Autodesk Fusion 360 part; units mm, degrees
(part 3 of 5)
sketch "midlayer" plane through (0, 0, 0) normal (0, 0, -1) x (1, 0, 0)
  line L0 (154.732, -58.8215) -> (154.732, -59.8219)
  line L1 (154.732, -59.8219) -> (140.732, -59.8219)
  line L2 (140.732, -59.8219) -> (140.732, -58.8215)
  line L3 (140.732, -58.8215) -> (139.931, -58.8215)
  line L4 (139.931, -58.8215) -> (139.931, -55.7223)
  line L5 (139.931, -55.7223) -> (140.732, -55.7223)
  line L6 (140.732, -55.7223) -> (140.732, -49.9223)
  line L7 (140.732, -49.9223) -> (139.931, -49.9223)
  line L8 (139.931, -49.9223) -> (139.931, -46.8217)
  line L9 (139.931, -46.8217) -> (140.732, -46.8217)
  line L10 (140.732, -46.8217) -> (140.732, -45.8227)
  line L11 (140.732, -45.8227) -> (154.732, -45.8227)
  line L12 (154.732, -45.8227) -> (154.732, -46.8217)
  line L13 (154.732, -46.8217) -> (155.531, -46.8217)
  line L14 (155.531, -46.8217) -> (155.531, -49.9223)
  line L15 (155.531, -49.9223) -> (154.732, -49.9223)
  line L16 (154.732, -49.9223) -> (154.732, -55.7223)
  line L17 (154.732, -55.7223) -> (155.531, -55.7223)
  line L18 (155.531, -55.7223) -> (155.531, -58.8215)
  line L19 (155.531, -58.8215) -> (154.732, -58.8215)
  line L20 (116.632, -46.8217) -> (117.431, -46.8217)
  line L21 (117.431, -46.8217) -> (117.431, -49.9223)
  line L22 (117.431, -49.9223) -> (116.632, -49.9223)
  line L23 (116.632, -49.9223) -> (116.632, -55.7223)
  line L24 (116.632, -55.7223) -> (117.431, -55.7223)
  line L25 (117.431, -55.7223) -> (117.431, -58.8215)
  line L26 (117.431, -58.8215) -> (116.632, -58.8215)
  line L27 (116.632, -58.8215) -> (116.632, -59.8219)
  line L28 (116.632, -59.8219) -> (102.632, -59.8219)
  line L29 (102.632, -59.8219) -> (102.632, -58.8215)
  line L30 (102.632, -58.8215) -> (101.831, -58.8215)
  line L31 (101.831, -58.8215) -> (101.831, -55.7223)
  line L32 (101.831, -55.7223) -> (102.632, -55.7223)
  line L33 (102.632, -55.7223) -> (102.632, -49.9223)
  line L34 (102.632, -49.9223) -> (101.831, -49.9223)
  line L35 (101.831, -49.9223) -> (101.831, -46.8217)
  line L36 (101.831, -46.8217) -> (102.632, -46.8217)
  line L37 (102.632, -46.8217) -> (102.632, -45.8227)
  line L38 (102.632, -45.8227) -> (116.632, -45.8227)
  line L39 (116.632, -45.8227) -> (116.632, -46.8217)
  line L40 (192.832, -59.8219) -> (178.832, -59.8219)
  line L41 (178.832, -59.8219) -> (178.832, -58.8215)
  line L42 (178.832, -58.8215) -> (178.031, -58.8215)
  line L43 (178.031, -58.8215) -> (178.031, -55.7223)
  line L44 (178.031, -55.7223) -> (178.832, -55.7223)
  line L45 (178.832, -55.7223) -> (178.832, -49.9223)
  line L46 (178.832, -49.9223) -> (178.031, -49.9223)
  line L47 (178.031, -49.9223) -> (178.031, -46.8217)
  line L48 (178.031, -46.8217) -> (178.832, -46.8217)
  line L49 (178.832, -46.8217) -> (178.832, -45.8227)
  line L50 (178.832, -45.8227) -> (192.832, -45.8227)
  line L51 (192.832, -45.8227) -> (192.832, -46.8217)
  line L52 (192.832, -46.8217) -> (193.631, -46.8217)
  line L53 (193.631, -46.8217) -> (193.631, -49.9223)
  line L54 (193.631, -49.9223) -> (192.832, -49.9223)
  line L55 (192.832, -49.9223) -> (192.832, -55.7223)
  line L56 (192.832, -55.7223) -> (193.631, -55.7223)
  line L57 (193.631, -55.7223) -> (193.631, -58.8215)
  line L58 (193.631, -58.8215) -> (192.832, -58.8215)
  line L59 (192.832, -58.8215) -> (192.832, -59.8219)
  line L60 (76.1503, -36.6737) -> (76.9511, -36.6737)
  line L61 (76.9511, -36.6737) -> (76.9511, -39.7715)
  line L62 (76.9511, -39.7715) -> (76.1503, -39.7715)
  line L63 (76.1503, -39.7715) -> (76.1503, -40.7719)
  line L64 (76.1503, -40.7719) -> (62.151, -40.7719)
  line L65 (62.151, -40.7719) -> (62.151, -39.7715)
  line L66 (62.151, -39.7715) -> (61.3502, -39.7715)
  line L67 (61.3502, -39.7715) -> (61.3502, -36.6737)
  line L68 (61.3502, -36.6737) -> (62.151, -36.6737)
  line L69 (62.151, -36.6737) -> (62.151, -30.8722)
  line L70 (62.151, -30.8722) -> (61.3502, -30.8722)
  line L71 (61.3502, -30.8722) -> (61.3502, -27.7716)
  line L72 (61.3502, -27.7716) -> (62.151, -27.7716)
  line L73 (62.151, -27.7716) -> (62.151, -26.7725)
  line L74 (62.151, -26.7725) -> (76.1503, -26.7725)
  line L75 (76.1503, -26.7725) -> (76.1503, -27.7716)
  line L76 (76.1503, -27.7716) -> (76.9511, -27.7716)
  line L77 (76.9511, -27.7716) -> (76.9511, -30.8722)
  line L78 (76.9511, -30.8722) -> (76.1503, -30.8722)
  line L79 (76.1503, -30.8722) -> (76.1503, -36.6737)
  line L80 (130.919, -64.8727) -> (130.919, -65.8717)
  line L81 (130.919, -65.8717) -> (131.72, -65.8717)
  line L82 (131.72, -65.8717) -> (131.72, -68.9723)
  line L83 (131.72, -68.9723) -> (130.919, -68.9723)
  line L84 (130.919, -68.9723) -> (130.919, -74.7723)
  line L85 (130.919, -74.7723) -> (131.72, -74.7723)
  line L86 (131.72, -74.7723) -> (131.72, -77.8715)
  line L87 (131.72, -77.8715) -> (130.919, -77.8715)
  line L88 (130.919, -77.8715) -> (130.919, -78.8719)
  line L89 (130.919, -78.8719) -> (116.92, -78.8719)
  line L90 (116.92, -78.8719) -> (116.92, -77.8715)
  line L91 (116.92, -77.8715) -> (116.119, -77.8715)
  line L92 (116.119, -77.8715) -> (116.119, -74.7723)
  line L93 (116.119, -74.7723) -> (116.92, -74.7723)
  line L94 (116.92, -74.7723) -> (116.92, -68.9723)
  line L95 (116.92, -68.9723) -> (116.119, -68.9723)
  line L96 (116.119, -68.9723) -> (116.119, -65.8717)
  line L97 (116.119, -65.8717) -> (116.92, -65.8717)
  line L98 (116.92, -65.8717) -> (116.92, -64.8727)
  line L99 (116.92, -64.8727) -> (130.919, -64.8727)
  line L100 (169.019, -68.9723) -> (169.019, -74.7723)
  line L101 (169.019, -74.7723) -> (169.82, -74.7723)
  line L102 (169.82, -74.7723) -> (169.82, -77.8715)
  line L103 (169.82, -77.8715) -> (169.019, -77.8715)
  line L104 (169.019, -77.8715) -> (169.019, -78.8719)
  line L105 (169.019, -78.8719) -> (155.02, -78.8719)
  line L106 (155.02, -78.8719) -> (155.02, -77.8715)
  line L107 (155.02, -77.8715) -> (154.219, -77.8715)
  line L108 (154.219, -77.8715) -> (154.219, -74.7723)
  line L109 (154.219, -74.7723) -> (155.02, -74.7723)
  line L110 (155.02, -74.7723) -> (155.02, -68.9723)
  line L111 (155.02, -68.9723) -> (154.219, -68.9723)
  line L112 (154.219, -68.9723) -> (154.219, -65.8717)
  line L113 (154.219, -65.8717) -> (155.02, -65.8717)
  line L114 (155.02, -65.8717) -> (155.02, -64.8727)
  line L115 (155.02, -64.8727) -> (169.019, -64.8727)
  line L116 (169.019, -64.8727) -> (169.019, -65.8717)
  line L117 (169.019, -65.8717) -> (169.82, -65.8717)
  line L118 (169.82, -65.8717) -> (169.82, -68.9723)
  line L119 (169.82, -68.9723) -> (169.019, -68.9723)
  arc A0 (54.0504, -25.8024) -> (53.0504, -26.8024) centre (54.0504, -26.8024) ccw
  line L120 (54.0504, -25.8024) -> (59.6225, -25.8024)
  arc A1 (60.6225, -26.8024) -> (59.6225, -25.8024) centre (59.6225, -26.8024) ccw
  line L121 (60.6225, -26.8024) -> (60.6225, -38.3016)
  arc A2 (59.6225, -39.3016) -> (60.6225, -38.3016) centre (59.6225, -38.3016) ccw
  line L122 (59.6225, -39.3016) -> (54.0504, -39.3016)
  arc A3 (53.0504, -38.3016) -> (54.0504, -39.3016) centre (54.0504, -38.3016) ccw
  line L123 (53.0504, -38.3016) -> (53.0504, -26.8024)
  line L124 (219.025, -17.6237) -> (219.826, -17.6237)
  line L125 (219.826, -17.6237) -> (219.826, -20.7216)
  line L126 (219.826, -20.7216) -> (219.025, -20.7216)
  line L127 (219.025, -20.7216) -> (219.025, -21.722)
  line L128 (219.025, -21.722) -> (205.026, -21.722)
  line L129 (205.026, -21.722) -> (205.026, -20.7216)
  line L130 (205.026, -20.7216) -> (204.225, -20.7216)
  line L131 (204.225, -20.7216) -> (204.225, -17.6237)
  line L132 (204.225, -17.6237) -> (205.026, -17.6237)
  line L133 (205.026, -17.6237) -> (205.026, -11.8222)
  line L134 (205.026, -11.8222) -> (204.225, -11.8222)
  line L135 (204.225, -11.8222) -> (204.225, -8.7216)
  line L136 (204.225, -8.7216) -> (205.026, -8.7216)
  line L137 (205.026, -8.7216) -> (205.026, -7.7225)
  line L138 (205.026, -7.7225) -> (219.025, -7.7225)
  line L139 (219.025, -7.7225) -> (219.025, -8.7216)
  line L140 (219.025, -8.7216) -> (219.826, -8.7216)
  line L141 (219.826, -8.7216) -> (219.826, -11.8222)
  line L142 (219.826, -11.8222) -> (219.025, -11.8222)
  line L143 (219.025, -11.8222) -> (219.025, -17.6237)
  line L144 (150.77, -65.8717) -> (150.77, -68.9723)
  line L145 (150.77, -68.9723) -> (149.969, -68.9723)
  line L146 (149.969, -68.9723) -> (149.969, -74.7723)
  line L147 (149.969, -74.7723) -> (150.77, -74.7723)
  line L148 (150.77, -74.7723) -> (150.77, -77.8715)
  line L149 (150.77, -77.8715) -> (149.969, -77.8715)
  line L150 (149.969, -77.8715) -> (149.969, -78.8719)
  line L151 (149.969, -78.8719) -> (135.97, -78.8719)
  line L152 (135.97, -78.8719) -> (135.97, -77.8715)
  line L153 (135.97, -77.8715) -> (135.169, -77.8715)
  line L154 (135.169, -77.8715) -> (135.169, -74.7723)
  line L155 (135.169, -74.7723) -> (135.97, -74.7723)
  line L156 (135.97, -74.7723) -> (135.97, -68.9723)
  line L157 (135.97, -68.9723) -> (135.169, -68.9723)
  line L158 (135.169, -68.9723) -> (135.169, -65.8717)
  line L159 (135.169, -65.8717) -> (135.97, -65.8717)
  line L160 (135.97, -65.8717) -> (135.97, -64.8727)
  line L161 (135.97, -64.8727) -> (149.969, -64.8727)
  line L162 (149.969, -64.8727) -> (149.969, -65.8717)
  line L163 (149.969, -65.8717) -> (150.77, -65.8717)
  line L164 (119.725, -19.2517) -> (119.725, -7.7524)
  arc A4 (120.725, -6.7524) -> (119.725, -7.7524) centre (120.725, -7.7524) ccw
  line L165 (120.725, -6.7524) -> (131.063, -6.7524)
  arc A5 (132.063, -7.7524) -> (131.063, -6.7524) centre (131.063, -7.7524) ccw
  line L166 (132.063, -7.7524) -> (132.063, -19.2517)
  arc A6 (131.063, -20.2517) -> (132.063, -19.2517) centre (131.063, -19.2517) ccw
  line L167 (131.063, -20.2517) -> (120.725, -20.2517)
  arc A7 (119.725, -19.2517) -> (120.725, -20.2517) centre (120.725, -19.2517) ccw
  line L168 (307.132, -36.6723) -> (307.931, -36.6723)
  line L169 (307.931, -36.6723) -> (307.931, -39.7715)
  line L170 (307.931, -39.7715) -> (307.132, -39.7715)
  line L171 (307.132, -39.7715) -> (307.132, -40.7719)
  line L172 (307.132, -40.7719) -> (293.132, -40.7719)
  line L173 (293.132, -40.7719) -> (293.132, -39.7715)
  line L174 (293.132, -39.7715) -> (292.331, -39.7715)
  line L175 (292.331, -39.7715) -> (292.331, -36.6723)
  line L176 (292.331, -36.6723) -> (293.132, -36.6723)
  line L177 (293.132, -36.6723) -> (293.132, -30.8722)
  line L178 (293.132, -30.8722) -> (292.331, -30.8722)
  line L179 (292.331, -30.8722) -> (292.331, -27.7716)
  line L180 (292.331, -27.7716) -> (293.132, -27.7716)
  line L181 (293.132, -27.7716) -> (293.132, -26.7725)
  line L182 (293.132, -26.7725) -> (307.132, -26.7725)
  line L183 (307.132, -26.7725) -> (307.132, -27.7716)
  line L184 (307.132, -27.7716) -> (307.931, -27.7716)
  line L185 (307.931, -27.7716) -> (307.931, -30.8722)
  line L186 (307.931, -30.8722) -> (307.132, -30.8722)
  line L187 (307.132, -30.8722) -> (307.132, -36.6723)
  line L188 (185.688, -17.6237) -> (186.487, -17.6237)
  line L189 (186.487, -17.6237) -> (186.487, -20.7216)
  line L190 (186.487, -20.7216) -> (185.688, -20.7216)
  line L191 (185.688, -20.7216) -> (185.688, -21.722)
  line L192 (185.688, -21.722) -> (166.926, -21.722)
  line L193 (166.926, -21.722) -> (166.926, -20.7216)
  line L194 (166.926, -20.7216) -> (166.125, -20.7216)
  line L195 (166.125, -20.7216) -> (166.125, -17.6237)
  line L196 (166.125, -17.6237) -> (166.926, -17.6237)
  line L197 (166.926, -17.6237) -> (166.926, -11.8222)
  line L198 (166.926, -11.8222) -> (166.125, -11.8222)
  line L199 (166.125, -11.8222) -> (166.125, -8.7216)
  line L200 (166.125, -8.7216) -> (166.926, -8.7216)
  line L201 (166.926, -8.7216) -> (166.926, -7.7225)
  line L202 (166.926, -7.7225) -> (185.688, -7.7225)
  line L203 (185.688, -7.7225) -> (185.688, -8.7216)
  line L204 (185.688, -8.7216) -> (186.487, -8.7216)
  line L205 (186.487, -8.7216) -> (186.487, -11.8222)
  line L206 (186.487, -11.8222) -> (185.688, -11.8222)
  line L207 (185.688, -11.8222) -> (185.688, -17.6237)
  line L208 (147.588, -17.6237) -> (148.387, -17.6237)
  line L209 (148.387, -17.6237) -> (148.387, -20.7216)
  line L210 (148.387, -20.7216) -> (147.588, -20.7216)
  line L211 (147.588, -20.7216) -> (147.588, -21.722)
  line L212 (147.588, -21.722) -> (133.587, -21.722)
  line L213 (133.587, -21.722) -> (133.587, -20.7216)
  line L214 (133.587, -20.7216) -> (132.788, -20.7216)
  line L215 (132.788, -20.7216) -> (132.788, -17.6237)
  line L216 (132.788, -17.6237) -> (133.587, -17.6237)
  line L217 (133.587, -17.6237) -> (133.587, -11.8222)
  line L218 (133.587, -11.8222) -> (132.788, -11.8222)
  line L219 (132.788, -11.8222) -> (132.788, -8.7216)
  line L220 (132.788, -8.7216) -> (133.587, -8.7216)
  line L221 (133.587, -8.7216) -> (133.587, -7.7225)
  line L222 (133.587, -7.7225) -> (147.588, -7.7225)
  line L223 (147.588, -7.7225) -> (147.588, -8.7216)
  line L224 (147.588, -8.7216) -> (148.387, -8.7216)
  line L225 (148.387, -8.7216) -> (148.387, -11.8222)
  line L226 (148.387, -11.8222) -> (147.588, -11.8222)
  line L227 (147.588, -11.8222) -> (147.588, -17.6237)
  arc A8 (84.2847, -39.3016) -> (85.2847, -38.3016) centre (84.2847, -38.3016) ccw
  line L228 (84.2847, -39.3016) -> (78.676, -39.3016)
  arc A9 (77.676, -38.3016) -> (78.676, -39.3016) centre (78.676, -38.3016) ccw
  line L229 (77.676, -38.3016) -> (77.676, -26.8024)
  arc A10 (78.676, -25.8024) -> (77.676, -26.8024) centre (78.676, -26.8024) ccw
  line L230 (78.676, -25.8024) -> (84.2847, -25.8024)
  arc A11 (85.2847, -26.8024) -> (84.2847, -25.8024) centre (84.2847, -26.8024) ccw
  line L231 (85.2847, -26.8024) -> (85.2847, -38.3016)
  line L232 (97.8697, -65.8717) -> (97.8697, -64.8727)
  line L233 (97.8697, -64.8727) -> (111.869, -64.8727)
  line L234 (111.869, -64.8727) -> (111.869, -65.8717)
  line L235 (111.869, -65.8717) -> (112.67, -65.8717)
  line L236 (112.67, -65.8717) -> (112.67, -68.9723)
  line L237 (112.67, -68.9723) -> (111.869, -68.9723)
  line L238 (111.869, -68.9723) -> (111.869, -74.7723)
  line L239 (111.869, -74.7723) -> (112.67, -74.7723)
  line L240 (112.67, -74.7723) -> (112.67, -77.8715)
  line L241 (112.67, -77.8715) -> (111.869, -77.8715)
  line L242 (111.869, -77.8715) -> (111.869, -78.8719)
  line L243 (111.869, -78.8719) -> (97.8697, -78.8719)
  line L244 (97.8697, -78.8719) -> (97.8697, -77.8715)
  line L245 (97.8697, -77.8715) -> (97.0689, -77.8715)
  line L246 (97.0689, -77.8715) -> (97.0689, -74.7723)
  line L247 (97.0689, -74.7723) -> (97.8697, -74.7723)
  line L248 (97.8697, -74.7723) -> (97.8697, -68.9723)
  line L249 (97.8697, -68.9723) -> (97.0689, -68.9723)
  line L250 (97.0689, -68.9723) -> (97.0689, -65.8717)
  line L251 (97.0689, -65.8717) -> (97.8697, -65.8717)
  line L252 (212.17, -77.8715) -> (211.369, -77.8715)
  line L253 (211.369, -77.8715) -> (211.369, -74.7723)
  line L254 (211.369, -74.7723) -> (212.17, -74.7723)
  line L255 (212.17, -74.7723) -> (212.17, -68.9723)
  line L256 (212.17, -68.9723) -> (211.369, -68.9723)
  line L257 (211.369, -68.9723) -> (211.369, -65.8717)
  line L258 (211.369, -65.8717) -> (212.17, -65.8717)
  line L259 (212.17, -65.8717) -> (212.17, -64.8727)
  line L260 (212.17, -64.8727) -> (226.169, -64.8727)
  line L261 (226.169, -64.8727) -> (226.169, -65.8717)
  line L262 (226.169, -65.8717) -> (226.97, -65.8717)
  line L263 (226.97, -65.8717) -> (226.97, -68.9723)
  line L264 (226.97, -68.9723) -> (226.169, -68.9723)
  line L265 (226.169, -68.9723) -> (226.169, -74.7723)
  line L266 (226.169, -74.7723) -> (226.97, -74.7723)
  line L267 (226.97, -74.7723) -> (226.97, -77.8715)
  line L268 (226.97, -77.8715) -> (226.169, -77.8715)
  line L269 (226.169, -77.8715) -> (226.169, -78.8719)
  line L270 (226.169, -78.8719) -> (212.17, -78.8719)
  line L271 (212.17, -78.8719) -> (212.17, -77.8715)
  arc A12 (154.863, -20.2517) -> (155.863, -19.2517) centre (154.863, -19.2517) ccw
  line L272 (154.863, -20.2517) -> (150.112, -20.2517)
  arc A13 (149.112, -19.2517) -> (150.112, -20.2517) centre (150.112, -19.2517) ccw
  line L273 (149.112, -19.2517) -> (149.112, -7.7524)
  arc A14 (150.112, -6.7524) -> (149.112, -7.7524) centre (150.112, -7.7524) ccw
  line L274 (150.112, -6.7524) -> (154.863, -6.7524)
  arc A15 (155.863, -7.7524) -> (154.863, -6.7524) centre (154.863, -7.7524) ccw
  line L275 (155.863, -7.7524) -> (155.863, -19.2517)
  arc A16 (220.551, -19.2517) -> (221.551, -20.2517) centre (221.551, -19.2517) ccw
  line L276 (220.551, -19.2517) -> (220.551, -7.7524)
  arc A17 (221.551, -6.7524) -> (220.551, -7.7524) centre (221.551, -7.7524) ccw
  line L277 (221.551, -6.7524) -> (227.126, -6.7524)
  arc A18 (228.126, -7.7524) -> (227.126, -6.7524) centre (227.126, -7.7524) ccw
  line L278 (228.126, -7.7524) -> (228.126, -19.2517)
  arc A19 (227.126, -20.2517) -> (228.126, -19.2517) centre (227.126, -19.2517) ccw
  line L279 (227.126, -20.2517) -> (221.551, -20.2517)
  line L280 (284.032, -38.3016) -> (284.032, -26.8024)
  arc A20 (285.032, -25.8024) -> (284.032, -26.8024) centre (285.032, -26.8024) ccw
  line L281 (285.032, -25.8024) -> (290.607, -25.8024)
  arc A21 (291.607, -26.8024) -> (290.607, -25.8024) centre (290.607, -26.8024) ccw
  line L282 (291.607, -26.8024) -> (291.607, -38.3016)
  arc A22 (290.607, -39.3016) -> (291.607, -38.3016) centre (290.607, -38.3016) ccw
  line L283 (290.607, -39.3016) -> (285.032, -39.3016)
  arc A23 (284.032, -38.3016) -> (285.032, -39.3016) centre (285.032, -38.3016) ccw
  arc A24 (309.657, -25.8024) -> (308.657, -26.8024) centre (309.657, -26.8024) ccw
  line L284 (309.657, -25.8024) -> (315.248, -25.8024)
  arc A25 (316.248, -26.8024) -> (315.248, -25.8024) centre (315.248, -26.8024) ccw
  line L285 (316.248, -26.8024) -> (316.248, -38.3016)
  arc A26 (315.248, -39.3016) -> (316.248, -38.3016) centre (315.248, -38.3016) ccw
  line L286 (315.248, -39.3016) -> (309.657, -39.3016)
  arc A27 (308.657, -38.3016) -> (309.657, -39.3016) centre (309.657, -38.3016) ccw
  line L287 (308.657, -38.3016) -> (308.657, -26.8024)
  line L288 (319.038, -55.7223) -> (319.837, -55.7223)
  line L289 (319.837, -55.7223) -> (319.837, -58.8215)
  line L290 (319.837, -58.8215) -> (319.038, -58.8215)
  line L291 (319.038, -58.8215) -> (319.038, -59.8219)
  line L292 (319.038, -59.8219) -> (305.037, -59.8219)
  line L293 (305.037, -59.8219) -> (305.037, -58.8215)
  line L294 (305.037, -58.8215) -> (304.238, -58.8215)
  line L295 (304.238, -58.8215) -> (304.238, -55.7223)
  line L296 (304.238, -55.7223) -> (305.037, -55.7223)
  line L297 (305.037, -55.7223) -> (305.037, -49.9223)
  line L298 (305.037, -49.9223) -> (304.238, -49.9223)
  line L299 (304.238, -49.9223) -> (304.238, -46.8217)
  line L300 (304.238, -46.8217) -> (305.037, -46.8217)
  line L301 (305.037, -46.8217) -> (305.037, -45.8227)
  line L302 (305.037, -45.8227) -> (319.038, -45.8227)
  line L303 (319.038, -45.8227) -> (319.038, -46.8217)
  line L304 (319.038, -46.8217) -> (319.837, -46.8217)
  line L305 (319.837, -46.8217) -> (319.837, -49.9223)
  line L306 (319.837, -49.9223) -> (319.038, -49.9223)
  line L307 (319.038, -49.9223) -> (319.038, -55.7223)
  line L308 (303.513, -45.8525) -> (303.513, -57.3516)
  arc A28 (302.513, -58.3516) -> (303.513, -57.3516) centre (302.513, -57.3516) ccw
  line L309 (302.513, -58.3516) -> (296.938, -58.3516)
  arc A29 (295.938, -57.3516) -> (296.938, -58.3516) centre (296.938, -57.3516) ccw
  line L310 (295.938, -57.3516) -> (295.938, -45.8525)
  arc A30 (296.938, -44.8525) -> (295.938, -45.8525) centre (296.938, -45.8525) ccw
  line L311 (296.938, -44.8525) -> (302.513, -44.8525)
  arc A31 (303.513, -45.8525) -> (302.513, -44.8525) centre (302.513, -45.8525) ccw
  arc A32 (327.137, -58.3516) -> (328.137, -57.3516) centre (327.137, -57.3516) ccw
  line L312 (327.137, -58.3516) -> (321.562, -58.3516)
  arc A33 (320.562, -57.3516) -> (321.562, -58.3516) centre (321.562, -57.3516) ccw
  line L313 (320.562, -57.3516) -> (320.562, -45.8525)
  arc A34 (321.562, -44.8525) -> (320.562, -45.8525) centre (321.562, -45.8525) ccw
  line L314 (321.562, -44.8525) -> (327.137, -44.8525)
  arc A35 (328.137, -45.8525) -> (327.137, -44.8525) centre (327.137, -45.8525) ccw
  line L315 (328.137, -45.8525) -> (328.137, -57.3516)
  circle A36 centre (-4.6103, -105.1519) radius 1.55
  circle A37 centre (-4.6103, 4.27) radius 1.55
  circle A38 centre (371.512, -105.1519) radius 1.55
  circle A39 centre (371.512, 4.27) radius 1.55
  line L316 (174.07, -78.8719) -> (174.07, -77.8715)
  line L317 (174.07, -77.8715) -> (173.269, -77.8715)
  line L318 (173.269, -77.8715) -> (173.269, -74.7723)
  line L319 (173.269, -74.7723) -> (174.07, -74.7723)
  line L320 (174.07, -74.7723) -> (174.07, -68.9723)
  line L321 (174.07, -68.9723) -> (173.269, -68.9723)
  line L322 (173.269, -68.9723) -> (173.269, -65.8717)
  line L323 (173.269, -65.8717) -> (174.07, -65.8717)
  line L324 (174.07, -65.8717) -> (174.07, -64.8727)
  line L325 (174.07, -64.8727) -> (188.069, -64.8727)
  line L326 (188.069, -64.8727) -> (188.069, -65.8717)
  line L327 (188.069, -65.8717) -> (188.87, -65.8717)
  line L328 (188.87, -65.8717) -> (188.87, -68.9723)
  line L329 (188.87, -68.9723) -> (188.069, -68.9723)
  line L330 (188.069, -68.9723) -> (188.069, -74.7723)
  line L331 (188.069, -74.7723) -> (188.87, -74.7723)
  line L332 (188.87, -74.7723) -> (188.87, -77.8715)
  line L333 (188.87, -77.8715) -> (188.069, -77.8715)
  line L334 (188.069, -77.8715) -> (188.069, -78.8719)
  line L335 (188.069, -78.8719) -> (174.07, -78.8719)
  line L336 (207.119, -64.8727) -> (207.119, -65.8717)
  line L337 (207.119, -65.8717) -> (207.92, -65.8717)
  line L338 (207.92, -65.8717) -> (207.92, -68.9723)
  line L339 (207.92, -68.9723) -> (207.119, -68.9723)
  line L340 (207.119, -68.9723) -> (207.119, -74.7723)
  line L341 (207.119, -74.7723) -> (207.92, -74.7723)
  line L342 (207.92, -74.7723) -> (207.92, -77.8715)
  line L343 (207.92, -77.8715) -> (207.119, -77.8715)
  line L344 (207.119, -77.8715) -> (207.119, -78.8719)
  line L345 (207.119, -78.8719) -> (193.12, -78.8719)
  line L346 (193.12, -78.8719) -> (193.12, -77.8715)
  line L347 (193.12, -77.8715) -> (192.319, -77.8715)
  line L348 (192.319, -77.8715) -> (192.319, -74.7723)
  line L349 (192.319, -74.7723) -> (193.12, -74.7723)
  line L350 (193.12, -74.7723) -> (193.12, -68.9723)
  line L351 (193.12, -68.9723) -> (192.319, -68.9723)
  line L352 (192.319, -68.9723) -> (192.319, -65.8717)
  line L353 (192.319, -65.8717) -> (193.12, -65.8717)
  line L354 (193.12, -65.8717) -> (193.12, -64.8727)
  line L355 (193.12, -64.8727) -> (207.119, -64.8727)
  line L356 (182.794, -93.8223) -> (183.595, -93.8223)
  line L357 (183.595, -93.8223) -> (183.595, -88.0223)
  line L358 (183.595, -88.0223) -> (182.794, -88.0223)
  line L359 (182.794, -88.0223) -> (182.794, -84.9217)
  line L360 (182.794, -84.9217) -> (183.595, -84.9217)
  line L361 (183.595, -84.9217) -> (183.595, -83.9227)
  line L362 (183.595, -83.9227) -> (197.594, -83.9227)
  line L363 (197.594, -83.9227) -> (197.594, -84.9217)
  line L364 (197.594, -84.9217) -> (198.395, -84.9217)
  line L365 (198.395, -84.9217) -> (198.395, -88.0223)
  line L366 (198.395, -88.0223) -> (197.594, -88.0223)
  line L367 (197.594, -88.0223) -> (197.594, -93.8223)
  line L368 (197.594, -93.8223) -> (198.395, -93.8223)
  line L369 (198.395, -93.8223) -> (198.395, -96.9215)
  line L370 (198.395, -96.9215) -> (197.594, -96.9215)
  line L371 (197.594, -96.9215) -> (197.594, -97.9219)
  line L372 (197.594, -97.9219) -> (183.595, -97.9219)
  line L373 (183.595, -97.9219) -> (183.595, -96.9215)
  line L374 (183.595, -96.9215) -> (182.794, -96.9215)
  line L375 (182.794, -96.9215) -> (182.794, -93.8223)
  line L376 (201.844, -96.9215) -> (201.844, -93.8223)
  line L377 (201.844, -93.8223) -> (202.645, -93.8223)
  line L378 (202.645, -93.8223) -> (202.645, -88.0223)
  line L379 (202.645, -88.0223) -> (201.844, -88.0223)
  line L380 (201.844, -88.0223) -> (201.844, -84.9217)
  line L381 (201.844, -84.9217) -> (202.645, -84.9217)
  line L382 (202.645, -84.9217) -> (202.645, -83.9227)
  line L383 (202.645, -83.9227) -> (216.644, -83.9227)
  line L384 (216.644, -83.9227) -> (216.644, -84.9217)
  line L385 (216.644, -84.9217) -> (217.445, -84.9217)
  line L386 (217.445, -84.9217) -> (217.445, -88.0223)
  line L387 (217.445, -88.0223) -> (216.644, -88.0223)
  line L388 (216.644, -88.0223) -> (216.644, -93.8223)
  line L389 (216.644, -93.8223) -> (217.445, -93.8223)
  line L390 (217.445, -93.8223) -> (217.445, -96.9215)
  line L391 (217.445, -96.9215) -> (216.644, -96.9215)
  line L392 (216.644, -96.9215) -> (216.644, -97.9219)
  line L393 (216.644, -97.9219) -> (202.645, -97.9219)
  line L394 (202.645, -97.9219) -> (202.645, -96.9215)
  line L395 (202.645, -96.9215) -> (201.844, -96.9215)
  line L396 (220.894, -84.9217) -> (221.695, -84.9217)
  line L397 (221.695, -84.9217) -> (221.695, -83.9227)
  line L398 (221.695, -83.9227) -> (235.694, -83.9227)
  line L399 (235.694, -83.9227) -> (235.694, -84.9217)
  line L400 (235.694, -84.9217) -> (236.495, -84.9217)
  line L401 (236.495, -84.9217) -> (236.495, -88.0223)
  line L402 (236.495, -88.0223) -> (235.694, -88.0223)
  line L403 (235.694, -88.0223) -> (235.694, -93.8223)
  line L404 (235.694, -93.8223) -> (236.495, -93.8223)
  line L405 (236.495, -93.8223) -> (236.495, -96.9215)
  line L406 (236.495, -96.9215) -> (235.694, -96.9215)
  line L407 (235.694, -96.9215) -> (235.694, -97.9219)
  line L408 (235.694, -97.9219) -> (221.695, -97.9219)
  line L409 (221.695, -97.9219) -> (221.695, -96.9215)
  line L410 (221.695, -96.9215) -> (220.894, -96.9215)
  line L411 (220.894, -96.9215) -> (220.894, -93.8223)
  line L412 (220.894, -93.8223) -> (221.695, -93.8223)
  line L413 (221.695, -93.8223) -> (221.695, -88.0223)
  line L414 (221.695, -88.0223) -> (220.894, -88.0223)
  line L415 (220.894, -88.0223) -> (220.894, -84.9217)
  line L416 (254.744, -97.9219) -> (240.745, -97.9219)
  line L417 (240.745, -97.9219) -> (240.745, -96.9215)
  line L418 (240.745, -96.9215) -> (239.944, -96.9215)
  line L419 (239.944, -96.9215) -> (239.944, -93.8223)
  line L420 (239.944, -93.8223) -> (240.745, -93.8223)
  line L421 (240.745, -93.8223) -> (240.745, -88.0223)
  line L422 (240.745, -88.0223) -> (239.944, -88.0223)
  line L423 (239.944, -88.0223) -> (239.944, -84.9217)
  line L424 (239.944, -84.9217) -> (240.745, -84.9217)
  line L425 (240.745, -84.9217) -> (240.745, -83.9227)
  line L426 (240.745, -83.9227) -> (254.744, -83.9227)
  line L427 (254.744, -83.9227) -> (254.744, -84.9217)
  line L428 (254.744, -84.9217) -> (255.545, -84.9217)
  line L429 (255.545, -84.9217) -> (255.545, -88.0223)
  line L430 (255.545, -88.0223) -> (254.744, -88.0223)
  line L431 (254.744, -88.0223) -> (254.744, -93.8223)
  line L432 (254.744, -93.8223) -> (255.545, -93.8223)
  line L433 (255.545, -93.8223) -> (255.545, -96.9215)
  line L434 (255.545, -96.9215) -> (254.744, -96.9215)
  line L435 (254.744, -96.9215) -> (254.744, -97.9219)
  line L436 (144.694, -88.0223) -> (144.694, -84.9217)
  line L437 (144.694, -84.9217) -> (145.495, -84.9217)
  line L438 (145.495, -84.9217) -> (145.495, -83.9227)
  line L439 (145.495, -83.9227) -> (159.494, -83.9227)
  line L440 (159.494, -83.9227) -> (159.494, -84.9217)
  line L441 (159.494, -84.9217) -> (160.295, -84.9217)
  line L442 (160.295, -84.9217) -> (160.295, -88.0223)
  line L443 (160.295, -88.0223) -> (159.494, -88.0223)
  line L444 (159.494, -88.0223) -> (159.494, -93.8223)
  line L445 (159.494, -93.8223) -> (160.295, -93.8223)
  line L446 (160.295, -93.8223) -> (160.295, -96.9215)
  line L447 (160.295, -96.9215) -> (159.494, -96.9215)
  line L448 (159.494, -96.9215) -> (159.494, -97.9219)
  line L449 (159.494, -97.9219) -> (145.495, -97.9219)
  line L450 (145.495, -97.9219) -> (145.495, -96.9215)
  line L451 (145.495, -96.9215) -> (144.694, -96.9215)
  line L452 (144.694, -96.9215) -> (144.694, -93.8223)
  line L453 (144.694, -93.8223) -> (145.495, -93.8223)
  line L454 (145.495, -93.8223) -> (145.495, -88.0223)
  line L455 (145.495, -88.0223) -> (144.694, -88.0223)
  line L456 (164.545, -93.8223) -> (164.545, -88.0223)
  line L457 (164.545, -88.0223) -> (163.744, -88.0223)
  line L458 (163.744, -88.0223) -> (163.744, -84.9217)
  line L459 (163.744, -84.9217) -> (164.545, -84.9217)
  line L460 (164.545, -84.9217) -> (164.545, -83.9227)
  line L461 (164.545, -83.9227) -> (178.544, -83.9227)
  line L462 (178.544, -83.9227) -> (178.544, -84.9217)
  line L463 (178.544, -84.9217) -> (179.345, -84.9217)
  line L464 (179.345, -84.9217) -> (179.345, -88.0223)
  line L465 (179.345, -88.0223) -> (178.544, -88.0223)
  line L466 (178.544, -88.0223) -> (178.544, -93.8223)
  line L467 (178.544, -93.8223) -> (179.345, -93.8223)
  line L468 (179.345, -93.8223) -> (179.345, -96.9215)
  line L469 (179.345, -96.9215) -> (178.544, -96.9215)
  line L470 (178.544, -96.9215) -> (178.544, -97.9219)
  line L471 (178.544, -97.9219) -> (164.545, -97.9219)
  line L472 (164.545, -97.9219) -> (164.545, -96.9215)
  line L473 (164.545, -96.9215) -> (163.744, -96.9215)
  line L474 (163.744, -96.9215) -> (163.744, -93.8223)
  line L475 (163.744, -93.8223) -> (164.545, -93.8223)
  line L476 (258.994, -96.9215) -> (258.994, -93.8223)
  line L477 (258.994, -93.8223) -> (259.795, -93.8223)
  line L478 (259.795, -93.8223) -> (259.795, -88.0223)
  line L479 (259.795, -88.0223) -> (258.994, -88.0223)
  line L480 (258.994, -88.0223) -> (258.994, -84.9217)
  line L481 (258.994, -84.9217) -> (259.795, -84.9217)
  line L482 (259.795, -84.9217) -> (259.795, -83.9227)
  line L483 (259.795, -83.9227) -> (273.794, -83.9227)
  line L484 (273.794, -83.9227) -> (273.794, -84.9217)
  line L485 (273.794, -84.9217) -> (274.595, -84.9217)
  line L486 (274.595, -84.9217) -> (274.595, -88.0223)
  line L487 (274.595, -88.0223) -> (273.794, -88.0223)
  line L488 (273.794, -88.0223) -> (273.794, -93.8223)
  line L489 (273.794, -93.8223) -> (274.595, -93.8223)
  line L490 (274.595, -93.8223) -> (274.595, -96.9215)
  line L491 (274.595, -96.9215) -> (273.794, -96.9215)
  line L492 (273.794, -96.9215) -> (273.794, -97.9219)
  line L493 (273.794, -97.9219) -> (259.795, -97.9219)
  line L494 (259.795, -97.9219) -> (259.795, -96.9215)
  line L495 (259.795, -96.9215) -> (258.994, -96.9215)
  line L496 (278.044, -96.9215) -> (278.044, -93.8223)
  line L497 (278.044, -93.8223) -> (278.845, -93.8223)
  line L498 (278.845, -93.8223) -> (278.845, -88.0223)
  line L499 (278.845, -88.0223) -> (278.044, -88.0223)
  line L500 (278.044, -88.0223) -> (278.044, -84.9217)
  line L501 (278.044, -84.9217) -> (278.845, -84.9217)
  line L502 (278.845, -84.9217) -> (278.845, -83.9227)
  line L503 (278.845, -83.9227) -> (292.844, -83.9227)
  line L504 (292.844, -83.9227) -> (292.844, -84.9217)
  line L505 (292.844, -84.9217) -> (293.645, -84.9217)
  line L506 (293.645, -84.9217) -> (293.645, -88.0223)
  line L507 (293.645, -88.0223) -> (292.844, -88.0223)
  line L508 (292.844, -88.0223) -> (292.844, -93.8223)
  line L509 (292.844, -93.8223) -> (293.645, -93.8223)
  line L510 (293.645, -93.8223) -> (293.645, -96.9215)
  line L511 (293.645, -96.9215) -> (292.844, -96.9215)
  line L512 (292.844, -96.9215) -> (292.844, -97.9219)
  line L513 (292.844, -97.9219) -> (278.845, -97.9219)
  line L514 (278.845, -97.9219) -> (278.845, -96.9215)
  line L515 (278.845, -96.9215) -> (278.044, -96.9215)
  line L516 (364.282, -83.9227) -> (364.282, -84.9217)
  line L517 (364.282, -84.9217) -> (365.083, -84.9217)
  line L518 (365.083, -84.9217) -> (365.083, -88.0223)
  line L519 (365.083, -88.0223) -> (364.282, -88.0223)
  line L520 (364.282, -88.0223) -> (364.282, -93.8223)
  line L521 (364.282, -93.8223) -> (365.083, -93.8223)
  line L522 (365.083, -93.8223) -> (365.083, -96.9215)
  line L523 (365.083, -96.9215) -> (364.282, -96.9215)
  line L524 (364.282, -96.9215) -> (364.282, -97.9219)
  line L525 (364.282, -97.9219) -> (350.282, -97.9219)
  line L526 (350.282, -97.9219) -> (350.282, -96.9215)
  line L527 (350.282, -96.9215) -> (349.481, -96.9215)
  line L528 (349.481, -96.9215) -> (349.481, -93.8223)
  line L529 (349.481, -93.8223) -> (350.282, -93.8223)
  line L530 (350.282, -93.8223) -> (350.282, -88.0223)
  line L531 (350.282, -88.0223) -> (349.481, -88.0223)
  line L532 (349.481, -88.0223) -> (349.481, -84.9217)
  line L533 (349.481, -84.9217) -> (350.282, -84.9217)
  line L534 (350.282, -84.9217) -> (350.282, -83.9227)
  line L535 (350.282, -83.9227) -> (364.282, -83.9227)
  line L536 (2.6197, -68.9723) -> (1.819, -68.9723)
  line L537 (1.819, -68.9723) -> (1.819, -65.8717)
  line L538 (1.819, -65.8717) -> (2.6197, -65.8717)
  line L539 (2.6197, -65.8717) -> (2.6197, -64.8727)
  line L540 (2.6197, -64.8727) -> (16.6192, -64.8727)
  line L541 (16.6192, -64.8727) -> (16.6192, -65.8717)
  line L542 (16.6192, -65.8717) -> (17.4198, -65.8717)
  line L543 (17.4198, -65.8717) -> (17.4198, -68.9723)
  line L544 (17.4198, -68.9723) -> (16.6192, -68.9723)
  line L545 (16.6192, -68.9723) -> (16.6192, -74.7723)
  line L546 (16.6192, -74.7723) -> (17.4198, -74.7723)
  line L547 (17.4198, -74.7723) -> (17.4198, -77.8715)
  line L548 (17.4198, -77.8715) -> (16.6192, -77.8715)
  line L549 (16.6192, -77.8715) -> (16.6192, -78.8719)
  line L550 (16.6192, -78.8719) -> (2.6196, -78.8719)
  line L551 (2.6197, -78.8719) -> (2.6197, -77.8715)
  line L552 (2.6197, -77.8715) -> (1.819, -77.8715)
  line L553 (1.819, -77.8715) -> (1.819, -74.7723)
  line L554 (1.819, -74.7723) -> (2.6197, -74.7723)
  line L555 (2.6197, -74.7723) -> (2.6197, -68.9723)
  line L556 (330.944, -83.9227) -> (330.944, -84.9217)
  line L557 (330.944, -84.9217) -> (331.745, -84.9217)
  line L558 (331.745, -84.9217) -> (331.745, -88.0223)
  line L559 (331.745, -88.0223) -> (330.944, -88.0223)
  line L560 (330.944, -88.0223) -> (330.944, -93.8223)
  line L561 (330.944, -93.8223) -> (331.745, -93.8223)
  line L562 (331.745, -93.8223) -> (331.745, -96.9215)
  line L563 (331.745, -96.9215) -> (330.944, -96.9215)
  line L564 (330.944, -96.9215) -> (330.944, -97.9219)
  line L565 (330.944, -97.9219) -> (297.895, -97.9219)
  line L566 (297.895, -97.9219) -> (297.895, -96.9215)
  line L567 (297.895, -96.9215) -> (297.094, -96.9215)
  line L568 (297.094, -96.9215) -> (297.094, -93.8223)
  line L569 (297.094, -93.8223) -> (297.895, -93.8223)
  line L570 (297.895, -93.8223) -> (297.895, -88.0223)
  line L571 (297.895, -88.0223) -> (297.094, -88.0223)
  line L572 (297.094, -88.0223) -> (297.094, -84.9217)
  line L573 (297.094, -84.9217) -> (297.895, -84.9217)
  line L574 (297.895, -84.9217) -> (297.895, -83.9227)
  line L575 (297.895, -83.9227) -> (300.87, -83.9227)
  line L576 (300.87, -83.9227) -> (300.87, -82.9525)
  line L577 (300.87, -82.9525) -> (304.169, -82.9525)
  line L578 (304.169, -82.9525) -> (304.169, -83.9227)
  line L579 (304.169, -83.9227) -> (324.67, -83.9227)
  line L580 (324.67, -83.9227) -> (324.67, -82.9525)
  line L581 (324.67, -82.9525) -> (327.969, -82.9525)
  line L582 (327.969, -82.9525) -> (327.969, -83.9227)
  line L583 (327.969, -83.9227) -> (330.944, -83.9227)
  line L584 (36.4698, -77.8715) -> (35.669, -77.8715)
  line L585 (35.669, -77.8715) -> (35.669, -78.8719)
  line L586 (35.669, -78.8719) -> (21.6697, -78.8719)
  line L587 (21.6697, -78.8719) -> (21.6697, -77.8715)
  line L588 (21.6697, -77.8715) -> (20.869, -77.8715)
  line L589 (20.869, -77.8715) -> (20.869, -74.7723)
  line L590 (20.869, -74.7723) -> (21.6697, -74.7723)
  line L591 (21.6697, -74.7723) -> (21.6697, -68.9723)
  line L592 (21.6697, -68.9723) -> (20.869, -68.9723)
  line L593 (20.869, -68.9723) -> (20.869, -65.8717)
  line L594 (20.869, -65.8717) -> (21.6697, -65.8717)
  line L595 (21.6697, -65.8717) -> (21.6697, -64.8727)
  line L596 (21.6697, -64.8727) -> (35.669, -64.8727)
  line L597 (35.669, -64.8727) -> (35.669, -65.8717)
  line L598 (35.669, -65.8717) -> (36.4698, -65.8717)
  line L599 (36.4698, -65.8717) -> (36.4698, -68.9723)
  line L600 (36.4698, -68.9723) -> (35.669, -68.9723)
  line L601 (35.669, -68.9723) -> (35.669, -74.7723)
  line L602 (35.669, -74.7723) -> (36.4698, -74.7723)
  line L603 (36.4698, -74.7723) -> (36.4698, -77.8715)
  line L604 (55.0072, -78.8719) -> (55.0072, -77.8715)
  line L605 (55.0072, -77.8715) -> (54.2064, -77.8715)
  line L606 (54.2064, -77.8715) -> (54.2064, -74.7723)
  line L607 (54.2064, -74.7723) -> (55.0072, -74.7723)
  line L608 (55.0072, -74.7723) -> (55.0072, -68.9723)
  line L609 (55.0072, -68.9723) -> (54.2064, -68.9723)
  line L610 (54.2064, -68.9723) -> (54.2064, -65.8717)
  line L611 (54.2064, -65.8717) -> (55.0072, -65.8717)
  line L612 (55.0072, -65.8717) -> (55.0072, -64.8727)
  line L613 (55.0072, -64.8727) -> (69.0065, -64.8727)
  line L614 (69.0065, -64.8727) -> (69.0065, -65.8717)
  line L615 (69.0065, -65.8717) -> (69.8059, -65.8717)
  line L616 (69.8059, -65.8717) -> (69.8059, -68.9723)
  line L617 (69.8059, -68.9723) -> (69.0065, -68.9723)
  line L618 (69.0065, -68.9723) -> (69.0065, -74.7723)
  line L619 (69.0065, -74.7723) -> (69.8059, -74.7723)
  line L620 (69.8059, -74.7723) -> (69.8059, -77.8715)
  line L621 (69.8059, -77.8715) -> (69.0065, -77.8715)
  line L622 (69.0065, -77.8715) -> (69.0065, -78.8719)
  line L623 (69.0065, -78.8719) -> (55.0072, -78.8719)
  line L624 (78.8197, -78.8719) -> (78.8197, -77.8715)
  line L625 (78.8197, -77.8715) -> (78.0189, -77.8715)
  line L626 (78.0189, -77.8715) -> (78.0189, -74.7723)
  line L627 (78.0189, -74.7723) -> (78.8197, -74.7723)
  line L628 (78.8197, -74.7723) -> (78.8197, -68.9723)
  line L629 (78.8197, -68.9723) -> (78.0189, -68.9723)
  line L630 (78.0189, -68.9723) -> (78.0189, -65.8717)
  line L631 (78.0189, -65.8717) -> (78.8197, -65.8717)
  line L632 (78.8197, -65.8717) -> (78.8197, -64.8727)
  line L633 (78.8197, -64.8727) -> (92.819, -64.8727)
  line L634 (92.819, -64.8727) -> (92.819, -65.8717)
  line L635 (92.819, -65.8717) -> (93.6198, -65.8717)
  line L636 (93.6198, -65.8717) -> (93.6198, -68.9723)
  line L637 (93.6198, -68.9723) -> (92.819, -68.9723)
  line L638 (92.819, -68.9723) -> (92.819, -74.7723)
  line L639 (92.819, -74.7723) -> (93.6198, -74.7723)
  line L640 (93.6198, -74.7723) -> (93.6198, -77.8715)
  line L641 (93.6198, -77.8715) -> (92.819, -77.8715)
  line L642 (92.819, -77.8715) -> (92.819, -78.8719)
  line L643 (92.819, -78.8719) -> (78.8197, -78.8719)
  line L644 (188.357, -40.7719) -> (188.357, -39.7715)
  line L645 (188.357, -39.7715) -> (187.556, -39.7715)
  line L646 (187.556, -39.7715) -> (187.556, -36.6737)
  line L647 (187.556, -36.6737) -> (188.357, -36.6737)
  line L648 (188.357, -36.6737) -> (188.357, -30.8722)
  line L649 (188.357, -30.8722) -> (187.556, -30.8722)
  line L650 (187.556, -30.8722) -> (187.556, -27.7716)
  line L651 (187.556, -27.7716) -> (188.357, -27.7716)
  line L652 (188.357, -27.7716) -> (188.357, -26.7725)
  line L653 (188.357, -26.7725) -> (202.357, -26.7725)
  line L654 (202.357, -26.7725) -> (202.357, -27.7716)
  line L655 (202.357, -27.7716) -> (203.156, -27.7716)
  line L656 (203.156, -27.7716) -> (203.156, -30.8722)
  line L657 (203.156, -30.8722) -> (202.357, -30.8722)
  line L658 (202.357, -30.8722) -> (202.357, -36.6737)
  line L659 (202.357, -36.6737) -> (203.156, -36.6737)
  line L660 (203.156, -36.6737) -> (203.156, -39.7715)
  line L661 (203.156, -39.7715) -> (202.357, -39.7715)
  line L662 (202.357, -39.7715) -> (202.357, -40.7719)
  line L663 (202.357, -40.7719) -> (188.357, -40.7719)
  line L664 (326.47, -7.0597) -> (325.669, -7.0597)
  line L665 (325.669, -7.0597) -> (325.669, -3.9605)
  line L666 (325.669, -3.9605) -> (326.47, -3.9605)
  line L667 (326.47, -3.9605) -> (326.47, -2.96)
  line L668 (326.47, -2.96) -> (340.469, -2.96)
  line L669 (340.469, -2.96) -> (340.469, -3.9605)
  line L670 (340.469, -3.9605) -> (341.27, -3.9605)
  line L671 (341.27, -3.9605) -> (341.27, -7.0597)
  line L672 (341.27, -7.0597) -> (340.469, -7.0597)
  line L673 (340.469, -7.0597) -> (340.469, -12.8598)
  line L674 (340.469, -12.8598) -> (341.27, -12.8598)
  line L675 (341.27, -12.8598) -> (341.27, -15.9604)
  line L676 (341.27, -15.9604) -> (340.469, -15.9604)
  line L677 (340.469, -15.9604) -> (340.469, -16.9595)
  line L678 (340.469, -16.9595) -> (326.47, -16.9595)
  line L679 (326.47, -16.9595) -> (326.47, -15.9604)
  line L680 (326.47, -15.9604) -> (325.669, -15.9604)
  line L681 (325.669, -15.9604) -> (325.669, -12.8598)
  line L682 (325.669, -12.8598) -> (326.47, -12.8598)
  line L683 (326.47, -12.8598) -> (326.47, -7.0597)
  line L684 (221.407, -40.7719) -> (207.407, -40.7719)
  line L685 (207.407, -40.7719) -> (207.407, -39.7715)
  line L686 (207.407, -39.7715) -> (206.606, -39.7715)
  line L687 (206.606, -39.7715) -> (206.606, -36.6737)
  line L688 (206.606, -36.6737) -> (207.407, -36.6737)
  line L689 (207.407, -36.6737) -> (207.407, -30.8722)
  line L690 (207.407, -30.8722) -> (206.606, -30.8722)
  line L691 (206.606, -30.8722) -> (206.606, -27.7716)
  line L692 (206.606, -27.7716) -> (207.407, -27.7716)
  line L693 (207.407, -27.7716) -> (207.407, -26.7725)
  line L694 (207.407, -26.7725) -> (221.407, -26.7725)
  line L695 (221.407, -26.7725) -> (221.407, -27.7716)
  line L696 (221.407, -27.7716) -> (222.206, -27.7716)
  line L697 (222.206, -27.7716) -> (222.206, -30.8722)
  line L698 (222.206, -30.8722) -> (221.407, -30.8722)
  line L699 (221.407, -30.8722) -> (221.407, -36.6737)
  line L700 (221.407, -36.6737) -> (222.206, -36.6737)
  line L701 (222.206, -36.6737) -> (222.206, -39.7715)
  line L702 (222.206, -39.7715) -> (221.407, -39.7715)
  line L703 (221.407, -39.7715) -> (221.407, -40.7719)
  line L704 (345.52, -12.8598) -> (345.52, -7.0597)
  line L705 (345.52, -7.0597) -> (344.719, -7.0597)
  line L706 (344.719, -7.0597) -> (344.719, -3.9605)
  line L707 (344.719, -3.9605) -> (345.52, -3.9605)
  line L708 (345.52, -3.9605) -> (345.52, -2.96)
  line L709 (345.52, -2.96) -> (359.519, -2.96)
  line L710 (359.519, -2.96) -> (359.519, -3.9605)
  line L711 (359.519, -3.9605) -> (360.32, -3.9605)
  line L712 (360.32, -3.9605) -> (360.32, -7.0597)
  line L713 (360.32, -7.0597) -> (359.519, -7.0597)
  line L714 (359.519, -7.0597) -> (359.519, -12.8598)
  line L715 (359.519, -12.8598) -> (360.32, -12.8598)
  line L716 (360.32, -12.8598) -> (360.32, -15.9604)
  line L717 (360.32, -15.9604) -> (359.519, -15.9604)
  line L718 (359.519, -15.9604) -> (359.519, -16.9595)
  line L719 (359.519, -16.9595) -> (345.52, -16.9595)
  line L720 (345.52, -16.9595) -> (345.52, -15.9604)
  line L721 (345.52, -15.9604) -> (344.719, -15.9604)
  line L722 (344.719, -15.9604) -> (344.719, -12.8598)
  line L723 (344.719, -12.8598) -> (345.52, -12.8598)
  line L724 (184.106, -30.8722) -> (183.307, -30.8722)
  line L725 (183.307, -30.8722) -> (183.307, -36.6737)
  line L726 (183.307, -36.6737) -> (184.106, -36.6737)
  line L727 (184.106, -36.6737) -> (184.106, -39.7715)
  line L728 (184.106, -39.7715) -> (183.307, -39.7715)
  line L729 (183.307, -39.7715) -> (183.307, -40.7719)
  line L730 (183.307, -40.7719) -> (169.307, -40.7719)
  line L731 (169.307, -40.7719) -> (169.307, -39.7715)
  line L732 (169.307, -39.7715) -> (168.506, -39.7715)
  line L733 (168.506, -39.7715) -> (168.506, -36.6737)
  line L734 (168.506, -36.6737) -> (169.307, -36.6737)
  line L735 (169.307, -36.6737) -> (169.307, -30.8722)
  line L736 (169.307, -30.8722) -> (168.506, -30.8722)
  line L737 (168.506, -30.8722) -> (168.506, -27.7716)
  line L738 (168.506, -27.7716) -> (169.307, -27.7716)
  line L739 (169.307, -27.7716) -> (169.307, -26.7725)
  line L740 (169.307, -26.7725) -> (183.307, -26.7725)
  line L741 (183.307, -26.7725) -> (183.307, -27.7716)
  line L742 (183.307, -27.7716) -> (184.106, -27.7716)
  line L743 (184.106, -27.7716) -> (184.106, -30.8722)
  line L744 (149.456, -39.7715) -> (149.456, -36.6737)
  line L745 (149.456, -36.6737) -> (150.257, -36.6737)
  line L746 (150.257, -36.6737) -> (150.257, -30.8722)
  line L747 (150.257, -30.8722) -> (149.456, -30.8722)
  line L748 (149.456, -30.8722) -> (149.456, -27.7716)
  line L749 (149.456, -27.7716) -> (150.257, -27.7716)
  line L750 (150.257, -27.7716) -> (150.257, -26.7725)
  line L751 (150.257, -26.7725) -> (164.257, -26.7725)
  line L752 (164.257, -26.7725) -> (164.257, -27.7716)
  line L753 (164.257, -27.7716) -> (165.056, -27.7716)
  line L754 (165.056, -27.7716) -> (165.056, -30.8722)
  line L755 (165.056, -30.8722) -> (164.257, -30.8722)
  line L756 (164.257, -30.8722) -> (164.257, -36.6737)
  line L757 (164.257, -36.6737) -> (165.056, -36.6737)
  line L758 (165.056, -36.6737) -> (165.056, -39.7715)
  line L759 (165.056, -39.7715) -> (164.257, -39.7715)
  line L760 (164.257, -39.7715) -> (164.257, -40.7719)
  line L761 (164.257, -40.7719) -> (150.257, -40.7719)
  line L762 (150.257, -40.7719) -> (150.257, -39.7715)
  line L763 (150.257, -39.7715) -> (149.456, -39.7715)
  line L764 (245.219, -74.7723) -> (246.02, -74.7723)
  line L765 (246.02, -74.7723) -> (246.02, -77.8715)
  line L766 (246.02, -77.8715) -> (245.219, -77.8715)
  line L767 (245.219, -77.8715) -> (245.219, -78.8719)
  line L768 (245.219, -78.8719) -> (231.22, -78.8719)
  line L769 (231.22, -78.8719) -> (231.22, -77.8715)
  line L770 (231.22, -77.8715) -> (230.419, -77.8715)
  line L771 (230.419, -77.8715) -> (230.419, -74.7723)
  line L772 (230.419, -74.7723) -> (231.22, -74.7723)
  line L773 (231.22, -74.7723) -> (231.22, -68.9723)
  line L774 (231.22, -68.9723) -> (230.419, -68.9723)
  line L775 (230.419, -68.9723) -> (230.419, -65.8717)
  line L776 (230.419, -65.8717) -> (231.22, -65.8717)
  line L777 (231.22, -65.8717) -> (231.22, -64.8727)
  line L778 (231.22, -64.8727) -> (245.219, -64.8727)
  line L779 (245.219, -64.8727) -> (245.219, -65.8717)
  line L780 (245.219, -65.8717) -> (246.02, -65.8717)
  line L781 (246.02, -65.8717) -> (246.02, -68.9723)
  line L782 (246.02, -68.9723) -> (245.219, -68.9723)
  line L783 (245.219, -68.9723) -> (245.219, -74.7723)
  line L784 (250.27, -68.9723) -> (249.469, -68.9723)
  line L785 (249.469, -68.9723) -> (249.469, -65.8717)
  line L786 (249.469, -65.8717) -> (250.27, -65.8717)
  line L787 (250.27, -65.8717) -> (250.27, -64.8727)
  line L788 (250.27, -64.8727) -> (264.269, -64.8727)
  line L789 (264.269, -64.8727) -> (264.269, -65.8717)
  line L790 (264.269, -65.8717) -> (265.07, -65.8717)
  line L791 (265.07, -65.8717) -> (265.07, -68.9723)
  line L792 (265.07, -68.9723) -> (264.269, -68.9723)
  line L793 (264.269, -68.9723) -> (264.269, -74.7723)
  line L794 (264.269, -74.7723) -> (265.07, -74.7723)
  line L795 (265.07, -74.7723) -> (265.07, -77.8715)
  line L796 (265.07, -77.8715) -> (264.269, -77.8715)
  line L797 (264.269, -77.8715) -> (264.269, -78.8719)
  line L798 (264.269, -78.8719) -> (250.27, -78.8719)
  line L799 (250.27, -78.8719) -> (250.27, -77.8715)
  line L800 (250.27, -77.8715) -> (249.469, -77.8715)
  line L801 (249.469, -77.8715) -> (249.469, -74.7723)
  line L802 (249.469, -74.7723) -> (250.27, -74.7723)
  line L803 (250.27, -74.7723) -> (250.27, -68.9723)
  line L804 (284.12, -74.7723) -> (284.12, -77.8715)
  line L805 (284.12, -77.8715) -> (283.319, -77.8715)
  line L806 (283.319, -77.8715) -> (283.319, -78.8719)
  line L807 (283.319, -78.8719) -> (269.32, -78.8719)
  line L808 (269.32, -78.8719) -> (269.32, -77.8715)
  line L809 (269.32, -77.8715) -> (268.519, -77.8715)
  line L810 (268.519, -77.8715) -> (268.519, -74.7723)
  line L811 (268.519, -74.7723) -> (269.32, -74.7723)
  line L812 (269.32, -74.7723) -> (269.32, -68.9723)
  line L813 (269.32, -68.9723) -> (268.519, -68.9723)
  line L814 (268.519, -68.9723) -> (268.519, -65.8717)
  line L815 (268.519, -65.8717) -> (269.32, -65.8717)
  line L816 (269.32, -65.8717) -> (269.32, -64.8727)
  line L817 (269.32, -64.8727) -> (283.319, -64.8727)
  line L818 (283.319, -64.8727) -> (283.319, -65.8717)
  line L819 (283.319, -65.8717) -> (284.12, -65.8717)
  line L820 (284.12, -65.8717) -> (284.12, -68.9723)
  line L821 (284.12, -68.9723) -> (283.319, -68.9723)
  line L822 (283.319, -68.9723) -> (283.319, -74.7723)
  line L823 (283.319, -74.7723) -> (284.12, -74.7723)
  line L824 (326.47, -26.1097) -> (325.669, -26.1097)
  line L825 (325.669, -26.1097) -> (325.669, -23.0105)
  line L826 (325.669, -23.0105) -> (326.47, -23.0105)
  line L827 (326.47, -23.0105) -> (326.47, -22.01)
  line L828 (326.47, -22.01) -> (340.469, -22.01)
  line L829 (340.469, -22.01) -> (340.469, -23.0105)
  line L830 (340.469, -23.0105) -> (341.27, -23.0105)
  line L831 (341.27, -23.0105) -> (341.27, -26.1097)
  line L832 (341.27, -26.1097) -> (340.469, -26.1097)
  line L833 (340.469, -26.1097) -> (340.469, -31.9098)
  line L834 (340.469, -31.9098) -> (341.27, -31.9098)
  line L835 (341.27, -31.9098) -> (341.27, -35.0104)
  line L836 (341.27, -35.0104) -> (340.469, -35.0104)
  line L837 (340.469, -35.0104) -> (340.469, -36.0094)
  line L838 (340.469, -36.0094) -> (326.47, -36.0094)
  line L839 (326.47, -36.0094) -> (326.47, -35.0104)
  line L840 (326.47, -35.0104) -> (325.669, -35.0104)
  line L841 (325.669, -35.0104) -> (325.669, -31.9098)
  line L842 (325.669, -31.9098) -> (326.47, -31.9098)
  line L843 (326.47, -31.9098) -> (326.47, -26.1097)
  line L844 (2.6197, -21.722) -> (2.6197, -20.7216)
  line L845 (2.6197, -20.7216) -> (1.819, -20.7216)
  line L846 (1.819, -20.7216) -> (1.819, -17.6237)
  line L847 (1.819, -17.6237) -> (2.6197, -17.6237)
  line L848 (2.6197, -17.6237) -> (2.6197, -11.8222)
  line L849 (2.6197, -11.8222) -> (1.819, -11.8222)
  line L850 (1.819, -11.8222) -> (1.819, -8.7216)
  line L851 (1.819, -8.7216) -> (2.6197, -8.7216)
  line L852 (2.6197, -8.7216) -> (2.6197, -7.7225)
  line L853 (2.6197, -7.7225) -> (16.6192, -7.7225)
  line L854 (16.6192, -7.7225) -> (16.6192, -8.7216)
  line L855 (16.6192, -8.7216) -> (17.4198, -8.7216)
  line L856 (17.4198, -8.7216) -> (17.4198, -11.8222)
  line L857 (17.4198, -11.8222) -> (16.6192, -11.8222)
  line L858 (16.6192, -11.8222) -> (16.6192, -17.6237)